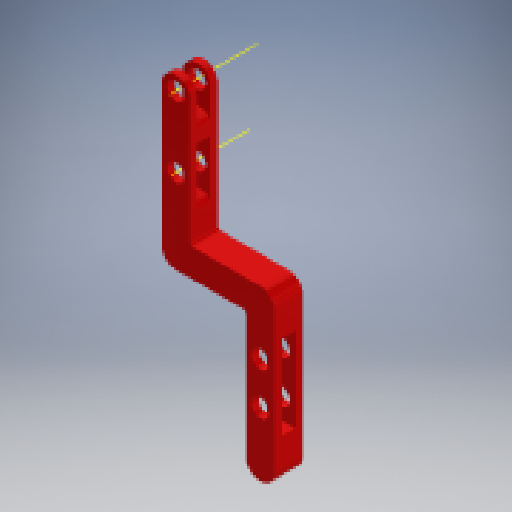
# Autodesk Inventor part: link7
Saved by Autodesk Inventor 2024.1 (Build 281209000, 209)
## iProperties
Created: 2023-09-09
Part Number: link7
Material: Aluminum 6061
Document SubType Name: Modeling
Designer: Camilo
Density: 2.7 g/cm^3
Appearance: Aluminum - Flat
Mass: 1.91312 g
Surface Area: 10.6958 cm^2
Volume: 0.708564 cm^3
Author: Camilo
Autodesk Inventor part; units mm, degrees
ref_plane "YZ Plane" through (0, 0, 0) normal (1, 0, 0) x (0, 1, 0)
ref_plane "XZ Plane" through (0, 0, 0) normal (0, 1, 0) x (-1, 0, 0)
ref_plane "XY Plane" through (0, 0, 0) normal (0, 0, 1) x (1, 0, 0)
sketch "Sketch1" plane through (0, 0, 0) normal (0, 0, 1) x (1, 0, 0)
  line L0 (0, 0) -> (4, 0)
  line L1 (4, 0) -> (4, -20)
  line L2 (0, 0) -> (-8, 0)
  line L3 (-8, 0) -> (-8, 20)
  circle A0 centre (-8, 20) radius 2
  circle A1 centre (-8, 20) radius 1.25
  line L4 (-8, 0) -> (-8, 10)
  circle A2 centre (-8, 10) radius 1.25
  circle A3 centre (4, 0) radius 2
  circle A4 centre (-8, 0) radius 2
  line L5 (-10, 20) -> (-10, 0)
  line L6 (-6, 20) -> (-6, 2.5)
  line L7 (-8, -2) -> (1.5, -2)
  line L8 (-5.5, 2) -> (4, 2)
  circle A5 centre (4, -20) radius 2
  line L9 (2, -20) -> (2, -2.5)
  line L10 (6, 0) -> (6, -20)
  arc A6 (-6, 2.5) -> (-5.5, 2) centre (-5.5, 2.5) ccw
  arc A7 (2, -2.5) -> (1.5, -2) centre (1.5, -2.5) ccw
  line L11 (-10, 20) -> (-6, 20)
  line L12 (-6, 20) -> (-6, 16)
  line L13 (-6, 16) -> (-10, 16)
  line L14 (-10, 16) -> (-10, 20)
  arc A8 (-6, 16) -> (-10, 16) centre (-8, 13.7639) ccw
  line L15 (-6, 10) -> (-10, 10)
  line L16 (-10, 10) -> (-10, 14)
  line L17 (-10, 14) -> (-6, 14)
  line L18 (-6, 14) -> (-6, 10)
  line L19 (-6, 10) -> (-10, 10)
  line L20 (-10, 10) -> (-10, 6)
  line L21 (-10, 6) -> (-6, 6)
  line L22 (-6, 6) -> (-6, 10)
  arc A9 (-10, 14) -> (-6, 14) centre (-8, 16.2361) ccw
  arc A10 (-6, 6) -> (-10, 6) centre (-8, 3.7639) ccw
  line L23 (4, 0) -> (4, -7)
  circle A11 centre (4, -7) radius 1.25
  line L24 (4, -20) -> (4, -13)
  circle A12 centre (4, -13) radius 1.25
  line L25 (2, -6.5) -> (2, -3.5)
  line L26 (6, -3.5) -> (6, -6.5)
  line L27 (2, -13.5) -> (2, -16.5)
  line L28 (6, -16.5) -> (6, -13.5)
  line L29 (6, -7) -> (2, -7)
  line L30 (2, -7) -> (2, -4)
  line L31 (2, -4) -> (6, -4)
  line L32 (6, -4) -> (6, -7)
  line L33 (6, -13) -> (2, -13)
  line L34 (2, -13) -> (2, -16)
  line L35 (2, -16) -> (6, -16)
  line L36 (6, -16) -> (6, -13)
  point P0 (-6, 0)
  point P1 (4, -2)
  point P2 (-8, 2)
  point P3 (4, 2)
  point P4 (2, 0)
  point P5 (2, -4)
  point P6 (2, -16)
  point P7 (6, -16)
  point P8 (6, -4)
  dimension "d44" = 4
  dimension "d45" = 20
  dimension "d46" = 8
  dimension "d47" = 20
  dimension "d48" = 4
  dimension "d49" = 2.5
  dimension "d50" = 10
  dimension "d51" = 2.5
  dimension "d52" = 4
  dimension "d53" = 4
  dimension "d54" = 4
  dimension "d55" = 0.5
  dimension "d56" = 0.5
  dimension "d57" = 4
  dimension "d58" = 20
  dimension "d59" = 3
  dimension "d60" = 4
  dimension "d61" = 10
  dimension "d62" = 4
  dimension "d63" = 3
  dimension "d64" = 3
  dimension "d66" = 2.5
  dimension "d68" = 2.5
  dimension "d75" = 7
  dimension "d77" = 7
  dimension "d78" = 3
  dimension "d79" = 3
  constraints: 74 end point, 23 point on circle, 21 point on line, 13 centre point, 13 parallel, 8 coincident, 7 horizontal, 7 perpendicular, 6 tangent, 2 midpoint
  measures "d44" distance of L0.start L0.end
  measures "d45" distance of L0.end L1.end
  measures "d46" distance of L0.start L2.end
  measures "d47" distance of L2.end L3.end
  measures "d48" diameter of A0
  measures "d49" diameter of A1
  measures "d50" distance of L2.end L4.end
  measures "d51" diameter of A2
  measures "d52" diameter of A3
  measures "d53" diameter of A4
  measures "d54" diameter of A5
  measures "d55" radius of A6
  measures "d56" radius of A7
  measures "d57" distance of L11.end L12.end
  measures "d58" distance of L5.start L5.end
  measures "d59" radius of A8
  measures "d60" distance of L15.end L16.end
  measures "d61" distance from line of L15 L5.end
  measures "d62" distance of L20.end L19.end
  measures "d63" radius of A9
  measures "d64" radius of A10
  measures "d66" diameter of A11
  measures "d68" diameter of A12
  measures "d75" distance of A12.centre L24.start
  measures "d77" vertical distance of A11.centre L10.start
  measures "d78" distance of L29.end L30.end
  measures "d79" distance of L34.end L33.end
extrude "Extrusion8" add sketch "Sketch1" along normal mid plane 4 contours L2 A4 L3 L21 L6 A6 L8 A3 L0 | L0 A3 L1 L31 L9 A7 L7 A4 L2 | A3 L1 L0 | L0 L1 A3 | A4 L3 L2 | L2 L3 A4 | A3 L10 L31 L1 | A4 L5 L21 L3 | L31 L10 L29 A11 L1 | L1 A11 L29 L9 L31 | L21 A10 L3 | L3 A10 L21 | L5 L15 A2 L3 A10 | L3 A2 L15 L6 A10 | L29 L10 L33 A12 L1 A11 | A11 L1 A12 L33 L9 L29 | L5 A9 L3 A2 L15 | L15 A2 L3 A9 L6 | L5 L13 L3 L17 | L17 L3 A9 | L17 L3 L13 L6 | A9 L3 L17 | L10 L35 L1 A12 L33 | L33 A12 L1 L35 L9 | A8 L3 L13 | L5 A0 L3 A8 | A8 L3 A0 L6 | L13 L3 A8 | L11 A1 L3 A0 | A0 L11 A1 | A0 L3 A1 L11 | L10 A5 L1 L35 | L35 L1 A5 L9 | A5
extrude "Extrusion9" cut sketch "Sketch1" along normal mid plane 2 contours L31 L10 L29 A11 L1 | L1 A11 L29 L9 L31 | L5 L15 A2 L3 A10 | L3 A2 L15 L6 A10 | L29 L10 L33 A12 L1 A11 | A11 L1 A12 L33 L9 L29 | L5 A9 L3 A2 L15 | L15 A2 L3 A9 L6 | L10 L35 L1 A12 L33 | L33 A12 L1 L35 L9 | L5 A0 L3 A8 | A8 L3 A0 L6 | L11 A1 L3 A0 | A0 L11 A1 | A0 L3 A1 L11
body "Solid3"
